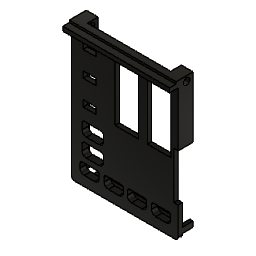
v2 - Timer - Bottom overlay (Autodesk Fusion 360 design; units mm, degrees)
Autodesk Fusion 360 part; units mm, degrees
sketch "Sketch1" plane through (0, 0, 0) normal (0, 1, 0) x (1, 0, 0)
  line L0 (0, 0) -> (50, 0)
  line L1 (50, 0) -> (50, -63)
  line L2 (50, -63) -> (0, -63)
  line L3 (0, -63) -> (0, 0)
  line L4 (20.9, -55.9) -> (31, -55.9)
  line L5 (31, -55.9) -> (31, -30.5)
  line L6 (31, -30.5) -> (20.9, -30.5)
  line L7 (20.9, -30.5) -> (20.9, -55.9)
  line L8 (36, -55.9) -> (46.1, -55.9)
  line L9 (46.1, -55.9) -> (46.1, -30.5)
  line L10 (46.1, -30.5) -> (36, -30.5)
  line L11 (36, -30.5) -> (36, -55.9)
  line L12 (0, 0) -> (50, 0)
  line L13 (50, 0) -> (50, 2)
  line L14 (50, 2) -> (0, 2)
  line L15 (0, 2) -> (0, 0)
  line L16 (6, -32.5) -> (11, -32.5)
  line L17 (11, -32.5) -> (11, -30.5)
  line L18 (11, -30.5) -> (6, -30.5)
  line L19 (6, -30.5) -> (6, -32.5)
  line L20 (6, -44.2) -> (11, -44.2)
  line L21 (11, -44.2) -> (11, -42.2)
  line L22 (11, -42.2) -> (6, -42.2)
  line L23 (6, -42.2) -> (6, -44.2)
  line L24 (6, -55.9) -> (11, -55.9)
  line L25 (11, -55.9) -> (11, -53.9)
  line L26 (11, -53.9) -> (6, -53.9)
  line L27 (6, -53.9) -> (6, -55.9)
  line L28 (13, -2.5) -> (4, -2.5)
  line L29 (4, -2.5) -> (4, -7.5)
  line L30 (4, -7.5) -> (13, -7.5)
  line L31 (13, -7.5) -> (13, -2.5)
  line L32 (13, -2.5) -> (4, -7.5) construction
  line L33 (4, -2.5) -> (13, -7.5) construction
  line L34 (24.33, -2.5) -> (15.33, -2.5)
  line L35 (15.33, -2.5) -> (15.33, -7.5)
  line L36 (15.33, -7.5) -> (24.33, -7.5)
  line L37 (24.33, -7.5) -> (24.33, -2.5)
  line L38 (24.33, -2.5) -> (15.33, -7.5) construction
  line L39 (15.33, -2.5) -> (24.33, -7.5) construction
  line L40 (35.16, -2.5) -> (26.16, -2.5)
  line L41 (26.16, -2.5) -> (26.16, -7.5)
  line L42 (26.16, -7.5) -> (35.16, -7.5)
  line L43 (35.16, -7.5) -> (35.16, -2.5)
  line L44 (35.16, -2.5) -> (26.16, -7.5) construction
  line L45 (26.16, -2.5) -> (35.16, -7.5) construction
  line L46 (46.49, -2.5) -> (37.49, -2.5)
  line L47 (37.49, -2.5) -> (37.49, -7.5)
  line L48 (37.49, -7.5) -> (46.49, -7.5)
  line L49 (46.49, -7.5) -> (46.49, -2.5)
  line L50 (46.49, -2.5) -> (37.49, -7.5) construction
  line L51 (37.49, -2.5) -> (46.49, -7.5) construction
  line L52 (7, -24.5) -> (13, -24.5)
  line L53 (13, -18.5) -> (7, -18.5)
  line L54 (15, -18.5) -> (5, -18.5)
  line L55 (5, -18.5) -> (5, -24.5)
  line L56 (5, -24.5) -> (15, -24.5)
  line L57 (15, -24.5) -> (15, -18.5)
  line L58 (15, -18.5) -> (5, -24.5) construction
  line L59 (5, -18.5) -> (15, -24.5) construction
  line L60 (15, -10) -> (5, -10)
  line L61 (5, -10) -> (5, -16)
  line L62 (5, -16) -> (15, -16)
  line L63 (15, -16) -> (15, -10)
  line L64 (15, -10) -> (5, -16) construction
  line L65 (5, -10) -> (15, -16) construction
  point P0 (8.5, -5)
  point P1 (19.83, -5)
  point P2 (30.66, -5)
  point P3 (41.99, -5)
  point P4 (10, -21.5)
  point P5 (10, -13)
  dimension "d1" = 50
  dimension "d2" = 63
  dimension "d3" = 10.1
  dimension "d4" = 25.4
  dimension "d5" = 10.1
  dimension "d6" = 25.4
  dimension "d7" = 3.9
  dimension "d8" = 5
  dimension "d9" = 30.5
  dimension "d10" = 30.5
  dimension "d19" = 2
  dimension "d58" = 5
  dimension "d59" = 2
  dimension "d60" = 6
  dimension "d61" = 30.5
  dimension "d62" = 5
  dimension "d63" = 2
  dimension "d64" = 9.7
  dimension "d65" = 5
  dimension "d66" = 2
  dimension "d67" = 9.7
  dimension "d105" = 9
  dimension "d106" = 5
  dimension "d107" = 9
  dimension "d108" = 5
  dimension "d127" = 9
  dimension "d128" = 5
  dimension "d129" = 9
  dimension "d130" = 5
  dimension "d151" = 6
  dimension "d152" = 6
  dimension "d159" = 10
  dimension "d160" = 6
  dimension "d161" = 10
  dimension "d162" = 6
  constraint horizontal L0
  constraint vertical L1
  constraint horizontal L2
  constraint vertical L3
  constraint coincident L0.start L3.end
  constraint horizontal L4
  constraint vertical L5
  constraint horizontal L6
  constraint vertical L7
  constraint horizontal L8
  constraint vertical L9
  constraint horizontal L10
  constraint vertical L11
  constraint horizontal L12
  constraint vertical L13
  constraint horizontal L14
  constraint vertical L15
  constraint horizontal L16
  constraint vertical L17
  constraint horizontal L18
  constraint vertical L19
  constraint horizontal L20
  constraint vertical L21
  constraint horizontal L22
  constraint vertical L23
  constraint horizontal L24
  constraint vertical L25
  constraint horizontal L26
  constraint vertical L27
  constraint horizontal L28
  constraint perpendicular L28 L29
  constraint parallel L28 L30
  constraint parallel L29 L31
  constraint coincident L32 P0
  constraint coincident L33 P0
  constraint horizontal L34
  constraint perpendicular L34 L35
  constraint parallel L34 L36
  constraint parallel L35 L37
  constraint coincident L38 P1
  constraint coincident L39 P1
  constraint horizontal L40
  constraint perpendicular L40 L41
  constraint parallel L40 L42
  constraint parallel L41 L43
  constraint coincident L44 P2
  constraint coincident L45 P2
  constraint horizontal L46
  constraint perpendicular L46 L47
  constraint parallel L46 L48
  constraint parallel L47 L49
  constraint coincident L50 P3
  constraint coincident L51 P3
  constraint horizontal L52
  constraint horizontal L53
  constraint horizontal L54
  constraint perpendicular L54 L55
  constraint parallel L54 L56
  constraint parallel L55 L57
  constraint coincident L58 P4
  constraint coincident L59 P4
  constraint horizontal L60
  constraint perpendicular L60 L61
  constraint parallel L60 L62
  constraint parallel L61 L63
  constraint coincident L64 P5
  constraint coincident L65 P5
  measures "d1" distance of L0.start L0.end
  measures "d2" distance of L0.start L2.end
  measures "d3" distance of L4.start L4.end
  measures "d4" distance of L4.start L6.end
  measures "d5" distance of L8.start L8.end
  measures "d6" distance of L8.start L10.end
  measures "d7" distance of L1 L9
  measures "d8" distance of L5 L11
  measures "d9" distance of L0 L10
  measures "d10" distance of L0 L6
  measures "d19" distance of L0.start L14.end
  measures "d58" distance of L16.start L16.end
  measures "d59" distance of L16.start L18.end
  measures "d60" distance of L3 L19
  measures "d61" distance of L0 L18
  measures "d62" distance of L20.start L20.end
  measures "d63" distance of L20.start L22.end
  measures "d64" distance of L16 L22
  measures "d65" distance of L24.start L24.end
  measures "d66" distance of L24.start L26.end
  measures "d67" distance of L20 L26
  measures "d105" distance of L29.end L30.end
  measures "d106" distance of L28.end L29.end
  measures "d107" distance of L35.end L36.end
  measures "d108" distance of L34.end L35.end
  measures "d127" distance of L41.end L42.end
  measures "d128" distance of L40.end L41.end
  measures "d129" distance of L47.end L48.end
  measures "d130" distance of L46.end L47.end
  measures "d151" distance of L52.start L52.end
  measures "d152" distance of L52.start L53.end
  measures "d159" distance of L55.end L56.end
  measures "d160" distance of L54.end L55.end
  measures "d161" distance of L61.end L62.end
  measures "d162" distance of L60.end L61.end
extrude "Extrude1" add sketch "Sketch1" against normal blind 2 contours L0 L1 L2 L3 L12 | L16 L17 L18 L19 | L20 L21 L22 L23 | L24 L25 L26 L27 | L28 L29 L30 L31 | L34 L35 L36 L37 | L40 L41 L42 L43 | L46 L47 L48 L49 | L52 L53 L54 L55 L56 L57 | L60 L61 L62 L63
extrude "Extrude3" add 1 faces at (16.6667, -0.6667, 0) along direction (0, 0, -1) blind 2
fillet "Fillet5" radius 1.5 1 edges at (0, -1, -2)
fillet "Fillet6" radius 1.5 1 edges at (50, -1, -2)
extrude "Extrude10" cut 1 faces at (27.6333, -0.6667, 30.5) along direction (0, 0, -1) blind 0.5
extrude "Extrude11" cut 1 faces at (31, -0.6667, 47.2667) along direction (1, 0, 0) blind 0.5
extrude "Extrude12" cut 1 faces at (42.7333, -0.6667, 30.5) along direction (0, 0, -1) blind 0.5
extrude "Extrude13" cut 1 faces at (46.1, -0.6667, 47.2667) along direction (1, 0, 0) blind 0.5
extrude "Extrude14" cut 1 faces at (20.9, -0.6667, 38.6333) along direction (-1, 0, 0) blind 0.5
extrude "Extrude15" cut 1 faces at (24.1, -1.3333, 55.9) along direction (0, 0, 1) blind 0.5
extrude "Extrude16" cut 1 faces at (39.5333, -0.6667, 55.9) along direction (0, 0, 1) blind 0.5
extrude "Extrude17" cut 1 faces at (36, -1.3333, 38.8) along direction (-1, 0, 0) blind 0.5
extrude "Extrude18" cut sketch "Sketch1" against normal blind 7 contours L16 L17 L18 L19 | L20 L21 L22 L23 | L24 L25 L26 L27
extrude "Extrude19" cut 1 faces at (7.6667, -0.6667, 55.9) along direction (0, 0, 1) blind 0.5
extrude "Extrude20" cut 1 faces at (6, -0.6667, 54.7333) along direction (-1, 0, 0) blind 0.5
extrude "Extrude21" cut 1 faces at (6, -0.6667, 42.8667) along direction (-1, 0, 0) blind 0.5
extrude "Extrude22" cut 1 faces at (7.6667, -0.6667, 32.5) along direction (0, 0, 1) blind 0.5
extrude "Extrude23" cut 1 faces at (6, -0.6667, 31.3333) along direction (-1, 0, 0) blind 0.5
extrude "Extrude24" cut 1 faces at (9.1667, -0.6667, 30.5) along direction (0, 0, -1) blind 0.5
extrude "Extrude25" cut 1 faces at (11, -1.3333, 32) along direction (1, 0, 0) blind 0.5
extrude "Extrude26" cut 1 faces at (9.1667, -0.6667, 42.2) along direction (0, 0, -1) blind 0.5
extrude "Extrude27" cut 1 faces at (11, -0.6667, 43.3667) along direction (1, 0, 0) blind 0.5
extrude "Extrude28" cut 1 faces at (9.1667, -0.6667, 53.9) along direction (0, 0, -1) blind 0.5
extrude "Extrude29" cut 1 faces at (11, -1.3333, 55.4) along direction (1, 0, 0) blind 0.5
extrude "Extrude30" cut sketch "Sketch1" against normal blind 3 contours L28 L29 L30 L31 | L34 L35 L36 L37
fillet "Fillet7" radius 1 1 edges at (4, -1, 7.5)
fillet "Fillet8" radius 1 1 edges at (13, -1, 7.5)
fillet "Fillet9" radius 2 1 edges at (13, -1, 2.5)
fillet "Fillet10" radius 2 1 edges at (4, -1, 2.5)
fillet "Fillet11" radius 1 1 edges at (15.33, -1, 7.5)
fillet "Fillet12" radius 1 1 edges at (24.33, -1, 7.5)
fillet "Fillet13" radius 2 1 edges at (24.33, -1, 2.5)
fillet "Fillet14" radius 2 1 edges at (15.33, -1, 2.5)
extrude "Extrude31" cut sketch "Sketch1" against normal blind 4 contours L40 L41 L42 L43 | L46 L47 L48 L49
fillet "Fillet15" radius 2 1 edges at (46.49, -1, 2.5)
fillet "Fillet16" radius 2 1 edges at (35.16, -1, 2.5)
fillet "Fillet17" radius 2 1 edges at (26.16, -1, 2.5)
fillet "Fillet18" radius 2 1 edges at (37.49, -1, 2.5)
fillet "Fillet19" radius 1 1 edges at (46.49, -1, 7.5)
fillet "Fillet20" radius 1 1 edges at (35.16, -1, 7.5)
fillet "Fillet21" radius 1 1 edges at (26.16, -1, 7.5)
fillet "Fillet22" radius 1 1 edges at (37.49, -1, 7.5)
extrude "Extrude32" cut 1 faces at (7.5, -1.3333, 44.2) along direction (0, 0, 1) blind 0.5
extrude "Extrude33" cut sketch "Sketch1" against normal blind 6 contours L52 L53 L54 L55 L56 L57 | L60 L61 L62 L63
fillet "Fillet23" radius 1 1 edges at (15, -1, 24.5)
fillet "Fillet24" radius 2 1 edges at (15, -1, 18.5)
fillet "Fillet25" radius 1 1 edges at (5, -1, 24.5)
fillet "Fillet26" radius 1 1 edges at (5, -1, 16)
fillet "Fillet27" radius 1 1 edges at (15, -1, 16)
fillet "Fillet28" radius 2 1 edges at (15, -1, 10)
fillet "Fillet29" radius 2 1 edges at (5, -1, 10)
fillet "Fillet30" radius 2 1 edges at (5, -1, 18.5)
sketch "Sketch2" plane through (0, 0, 0) normal (0, 1, 0) x (-1, 0, 0)
  line L0 (-7, 18.5) -> (-13, 18.5)
  arc A0 (-15, 20.5) -> (-13, 18.5) centre (-13, 20.5) ccw
  line L1 (-15, 20.5) -> (-15, 23.5)
  arc A1 (-14, 24.5) -> (-15, 23.5) centre (-14, 23.5) ccw
  line L2 (-14, 24.5) -> (-6, 24.5)
  arc A2 (-5, 23.5) -> (-6, 24.5) centre (-6, 23.5) ccw
  line L3 (-5, 23.5) -> (-5, 20.5)
  arc A3 (-7, 18.5) -> (-5, 20.5) centre (-7, 20.5) ccw
  line L4 (-7, 10) -> (-13, 10)
  arc A4 (-15, 12) -> (-13, 10) centre (-13, 12) ccw
  line L5 (-15, 12) -> (-15, 15)
  arc A5 (-14, 16) -> (-15, 15) centre (-14, 15) ccw
  line L6 (-14, 16) -> (-6, 16)
  arc A6 (-5, 15) -> (-6, 16) centre (-6, 15) ccw
  line L7 (-5, 15) -> (-5, 12)
  arc A7 (-7, 10) -> (-5, 12) centre (-7, 12) ccw
  line L8 (-5.5, 53.4) -> (-11.5, 53.4)
  line L9 (-11.5, 53.4) -> (-11.5, 56.4)
  line L10 (-11.5, 56.4) -> (-5.5, 56.4)
  line L11 (-5.5, 56.4) -> (-5.5, 53.4)
  line L12 (-11.5, 41.7) -> (-11.5, 44.7)
  line L13 (-11.5, 44.7) -> (-5.5, 44.7)
  line L14 (-5.5, 44.7) -> (-5.5, 41.7)
  line L15 (-5.5, 41.7) -> (-11.5, 41.7)
  line L16 (-5.5, 30) -> (-11.5, 30)
  line L17 (-11.5, 30) -> (-11.5, 33)
  line L18 (-11.5, 33) -> (-5.5, 33)
  line L19 (-5.5, 33) -> (-5.5, 30)
  line L20 (-46.6, 56.4) -> (-35.5, 56.4)
  line L21 (-35.5, 56.4) -> (-35.5, 30)
  line L22 (-35.5, 30) -> (-46.6, 30)
  line L23 (-46.6, 30) -> (-46.6, 56.4)
  line L24 (-31.5, 30) -> (-31.5, 56.4)
  line L25 (-31.5, 56.4) -> (-20.4, 56.4)
  line L26 (-20.4, 56.4) -> (-20.4, 30)
  line L27 (-20.4, 30) -> (-31.5, 30)
  arc A8 (-50, -0.5) -> (-48.5, -2) centre (-48.5, -0.5) ccw
  line L28 (-48.5, -2) -> (-1.5, -2)
  arc A9 (-1.5, -2) -> (0, -0.5) centre (-1.5, -0.5) ccw
  line L29 (0, -0.5) -> (0, 63)
  line L30 (0, 63) -> (-50, 63)
  line L31 (-50, 63) -> (-50, -0.5)
  line L32 (-6, 2.5) -> (-11, 2.5)
  arc A10 (-13, 4.5) -> (-11, 2.5) centre (-11, 4.5) ccw
  line L33 (-13, 4.5) -> (-13, 6.5)
  arc A11 (-12, 7.5) -> (-13, 6.5) centre (-12, 6.5) ccw
  line L34 (-12, 7.5) -> (-5, 7.5)
  arc A12 (-4, 6.5) -> (-5, 7.5) centre (-5, 6.5) ccw
  line L35 (-4, 6.5) -> (-4, 4.5)
  arc A13 (-6, 2.5) -> (-4, 4.5) centre (-6, 4.5) ccw
  line L36 (-17.33, 2.5) -> (-22.33, 2.5)
  arc A14 (-24.33, 4.5) -> (-22.33, 2.5) centre (-22.33, 4.5) ccw
  line L37 (-24.33, 4.5) -> (-24.33, 6.5)
  arc A15 (-23.33, 7.5) -> (-24.33, 6.5) centre (-23.33, 6.5) ccw
  line L38 (-23.33, 7.5) -> (-16.33, 7.5)
  arc A16 (-15.33, 6.5) -> (-16.33, 7.5) centre (-16.33, 6.5) ccw
  line L39 (-15.33, 6.5) -> (-15.33, 4.5)
  arc A17 (-17.33, 2.5) -> (-15.33, 4.5) centre (-17.33, 4.5) ccw
  line L40 (-28.16, 2.5) -> (-33.16, 2.5)
  arc A18 (-35.16, 4.5) -> (-33.16, 2.5) centre (-33.16, 4.5) ccw
  line L41 (-35.16, 4.5) -> (-35.16, 6.5)
  arc A19 (-34.16, 7.5) -> (-35.16, 6.5) centre (-34.16, 6.5) ccw
  line L42 (-34.16, 7.5) -> (-27.16, 7.5)
  arc A20 (-26.16, 6.5) -> (-27.16, 7.5) centre (-27.16, 6.5) ccw
  line L43 (-26.16, 6.5) -> (-26.16, 4.5)
  arc A21 (-28.16, 2.5) -> (-26.16, 4.5) centre (-28.16, 4.5) ccw
  line L44 (-39.49, 2.5) -> (-44.49, 2.5)
  arc A22 (-46.49, 4.5) -> (-44.49, 2.5) centre (-44.49, 4.5) ccw
  line L45 (-46.49, 4.5) -> (-46.49, 6.5)
  arc A23 (-45.49, 7.5) -> (-46.49, 6.5) centre (-45.49, 6.5) ccw
  line L46 (-45.49, 7.5) -> (-38.49, 7.5)
  arc A24 (-37.49, 6.5) -> (-38.49, 7.5) centre (-38.49, 6.5) ccw
  line L47 (-37.49, 6.5) -> (-37.49, 4.5)
  arc A25 (-39.49, 2.5) -> (-37.49, 4.5) centre (-39.49, 4.5) ccw
  line L48 (-50, 63) -> (-48.5, 63)
  line L49 (-48.5, 63) -> (-48.5, 0)
  line L50 (-48.5, 0) -> (-50, 0)
  line L51 (-50, 0) -> (-50, 63)
  line L52 (0, 63) -> (-1.5, 63)
  line L53 (-1.5, 63) -> (-1.5, 0)
  line L54 (-1.5, 0) -> (0, 0)
  line L55 (0, 0) -> (0, 63)
  dimension "d181" = 1.5
  dimension "d182" = 63
  dimension "d183" = 1.5
  dimension "d184" = 63
  constraint horizontal L48
  constraint vertical L49
  constraint horizontal L50
  constraint vertical L51
  constraint coincident L30.end L31.start
  constraint horizontal L52
  constraint vertical L53
  constraint horizontal L54
  constraint vertical L55
  constraint coincident L29.end L30.start
  measures "d181" distance of L30.end L48.end
  measures "d182" distance of L30.end L50.end
  measures "d183" distance of L29.end L52.end
  measures "d184" distance of L29.end L54.end
extrude "Extrude34" add sketch "Sketch2" along normal blind 3 contours L30 L31 L48 L49 L50 L51 | L29 L30 L52 L53 L54 L55
extrude "Extrude35" add 2 faces at (49.5, 3, 42) (0.5, 3, 21) along direction (0, 1, 0) blind 2
sketch "Sketch3" plane through (50, 0, 0) normal (1, 0, 0) x (0, 1, 0)
  line L0 (-2, -0.5) -> (0, -0.5)
  line L1 (0, -0.5) -> (0, 0)
  line L2 (0, 0) -> (5, 0)
  line L3 (5, 0) -> (5, 63)
  line L4 (5, 63) -> (-2, 63)
  line L5 (-2, 63) -> (-2, -0.5)
  circle A0 centre (2, 60.7) radius 1.5
  dimension "d189" = 2.3
  dimension "d190" = 3
  dimension "d203" = 3
  measures "d189" distance of L4 A0.centre
  measures "d190" distance of L3 A0.centre
  measures "d203" diameter of A0
extrude "Extrude36" cut sketch "Sketch3" against normal blind 50 contours A0
sketch "Sketch4" plane through (48.5, 0, 0) normal (-1, 0, 0) x (0, -1, 0)
  circle A0 centre (-2, 60.7) radius 1.5
  line L0 (0, 0) -> (0, 63)
  line L1 (0, 63) -> (-5, 63)
  line L2 (-5, 63) -> (-5, 0)
  line L3 (-5, 0) -> (0, 0)
sketch "Sketch5" plane through (0, -2, 0) normal (0, -1, 0) x (1, 0, 0)
  line L0 (13, 18.5) -> (7, 18.5)
  arc A0 (5, 20.5) -> (7, 18.5) centre (7, 20.5) ccw
  line L1 (5, 20.5) -> (5, 23.5)
  arc A1 (6, 24.5) -> (5, 23.5) centre (6, 23.5) ccw
  line L2 (6, 24.5) -> (14, 24.5)
  arc A2 (15, 23.5) -> (14, 24.5) centre (14, 23.5) ccw
  line L3 (15, 23.5) -> (15, 20.5)
  arc A3 (13, 18.5) -> (15, 20.5) centre (13, 20.5) ccw
  line L4 (13, 10) -> (7, 10)
  arc A4 (5, 12) -> (7, 10) centre (7, 12) ccw
  line L5 (5, 12) -> (5, 15)
  arc A5 (6, 16) -> (5, 15) centre (6, 15) ccw
  line L6 (6, 16) -> (14, 16)
  arc A6 (15, 15) -> (14, 16) centre (14, 15) ccw
  line L7 (15, 15) -> (15, 12)
  arc A7 (13, 10) -> (15, 12) centre (13, 12) ccw
  line L8 (11.5, 44.7) -> (11.5, 41.7)
  line L9 (11.5, 41.7) -> (5.5, 41.7)
  line L10 (5.5, 41.7) -> (5.5, 44.7)
  line L11 (5.5, 44.7) -> (11.5, 44.7)
  line L12 (44.49, 2.5) -> (39.49, 2.5)
  arc A8 (37.49, 4.5) -> (39.49, 2.5) centre (39.49, 4.5) ccw
  line L13 (37.49, 4.5) -> (37.49, 6.5)
  arc A9 (38.49, 7.5) -> (37.49, 6.5) centre (38.49, 6.5) ccw
  line L14 (38.49, 7.5) -> (45.49, 7.5)
  arc A10 (46.49, 6.5) -> (45.49, 7.5) centre (45.49, 6.5) ccw
  line L15 (46.49, 6.5) -> (46.49, 4.5)
  arc A11 (44.49, 2.5) -> (46.49, 4.5) centre (44.49, 4.5) ccw
  line L16 (33.16, 2.5) -> (28.16, 2.5)
  arc A12 (26.16, 4.5) -> (28.16, 2.5) centre (28.16, 4.5) ccw
  line L17 (26.16, 4.5) -> (26.16, 6.5)
  arc A13 (27.16, 7.5) -> (26.16, 6.5) centre (27.16, 6.5) ccw
  line L18 (27.16, 7.5) -> (34.16, 7.5)
  arc A14 (35.16, 6.5) -> (34.16, 7.5) centre (34.16, 6.5) ccw
  line L19 (35.16, 6.5) -> (35.16, 4.5)
  arc A15 (33.16, 2.5) -> (35.16, 4.5) centre (33.16, 4.5) ccw
  line L20 (22.33, 2.5) -> (17.33, 2.5)
  arc A16 (15.33, 4.5) -> (17.33, 2.5) centre (17.33, 4.5) ccw
  line L21 (15.33, 4.5) -> (15.33, 6.5)
  arc A17 (16.33, 7.5) -> (15.33, 6.5) centre (16.33, 6.5) ccw
  line L22 (16.33, 7.5) -> (23.33, 7.5)
  arc A18 (24.33, 6.5) -> (23.33, 7.5) centre (23.33, 6.5) ccw
  line L23 (24.33, 6.5) -> (24.33, 4.5)
  arc A19 (22.33, 2.5) -> (24.33, 4.5) centre (22.33, 4.5) ccw
  line L24 (11, 2.5) -> (6, 2.5)
  arc A20 (4, 4.5) -> (6, 2.5) centre (6, 4.5) ccw
  line L25 (4, 4.5) -> (4, 6.5)
  arc A21 (5, 7.5) -> (4, 6.5) centre (5, 6.5) ccw
  line L26 (5, 7.5) -> (12, 7.5)
  arc A22 (13, 6.5) -> (12, 7.5) centre (12, 6.5) ccw
  line L27 (13, 6.5) -> (13, 4.5)
  arc A23 (11, 2.5) -> (13, 4.5) centre (11, 4.5) ccw
  line L28 (11.5, 53.4) -> (5.5, 53.4)
  line L29 (5.5, 53.4) -> (5.5, 56.4)
  line L30 (5.5, 56.4) -> (11.5, 56.4)
  line L31 (11.5, 56.4) -> (11.5, 53.4)
  line L32 (11.5, 30) -> (5.5, 30)
  line L33 (5.5, 30) -> (5.5, 33)
  line L34 (5.5, 33) -> (11.5, 33)
  line L35 (11.5, 33) -> (11.5, 30)
  line L36 (35.5, 56.4) -> (46.6, 56.4)
  line L37 (46.6, 56.4) -> (46.6, 30)
  line L38 (46.6, 30) -> (35.5, 30)
  line L39 (35.5, 30) -> (35.5, 56.4)
  line L40 (31.5, 56.4) -> (31.5, 30)
  line L41 (31.5, 30) -> (20.4, 30)
  line L42 (20.4, 30) -> (20.4, 56.4)
  line L43 (20.4, 56.4) -> (31.5, 56.4)
  arc A24 (48.5, -2) -> (50, -0.5) centre (48.5, -0.5) ccw
  line L44 (50, -0.5) -> (50, 63)
  line L45 (50, 63) -> (0, 63)
  line L46 (0, 63) -> (0, -0.5)
  arc A25 (0, -0.5) -> (1.5, -2) centre (1.5, -0.5) ccw
  line L47 (1.5, -2) -> (48.5, -2)
  line L48 (0, 63) -> (50, 63)
  line L49 (50, 63) -> (50, 61)
  line L50 (50, 61) -> (0, 61)
  line L51 (0, 61) -> (0, 63)
  line L52 (0, 61) -> (50, 61)
  line L53 (50, 61) -> (50, 62)
  line L54 (50, 62) -> (0, 62)
  line L55 (0, 62) -> (0, 61)
  constraint horizontal L48
  constraint vertical L49
  constraint horizontal L50
  constraint vertical L51
  constraint coincident L44 L49.end
  constraint coincident L45.end L46.start
  constraint horizontal L52
  constraint vertical L53
  constraint horizontal L54
  constraint vertical L55
  constraint midpoint L49 L53.end
extrude "Extrude37" add sketch "Sketch5" along normal blind 3 contours L44 L46 L49 L50 L51 L52 L53 L54 L55
extrude "Extrude38" add 1 faces at (16.6667, -5, 61.3333) along direction (0, -1, 0) blind 1
extrude "Extrude39" add 1 faces at (33.3333, -4.6667, 61) along direction (0, 0, -1) blind 1
extrude "Extrude40" add 1 faces at (33.3333, -2, 62.3333) along direction (0, -1, 0) blind 1
sketch "Sketch6" plane through (1.5, 0, 0) normal (1, 0, 0) x (0, 1, 0)
  circle A0 centre (2, 60.7) radius 1.5
  line L0 (0, 63) -> (0, 0)
  line L1 (0, 0) -> (5, 0)
  line L2 (5, 0) -> (5, 63)
  line L3 (5, 63) -> (0, 63)
  line L4 (5, 63) -> (0, 63)
  line L5 (0, 63) -> (0, 58)
  line L6 (0, 58) -> (5, 58)
  line L7 (5, 58) -> (5, 63)
  dimension "d204" = 5
  constraint horizontal L4
  constraint vertical L5
  constraint horizontal L6
  constraint vertical L7
  constraint coincident L0 L5.end
  constraint coincident L2.end L3.start
  measures "d204" distance of L2.end L6.end
extrude "Extrude42" add sketch "Sketch6" along normal blind 48 contours L0 L2 L3 L4 L5 L6 L7
sketch "Sketch7" plane through (0, 5, 0) normal (0, 1, 0) x (-1, 0, 0)
  line L0 (0, 0) -> (0, 63)
  line L1 (0, 63) -> (-50, 63)
  line L2 (-50, 63) -> (-50, 0)
  line L3 (-50, 0) -> (-48.5, 0)
  line L4 (-48.5, 0) -> (-48.5, 58)
  line L5 (-48.5, 58) -> (-1.5, 58)
  line L6 (-1.5, 58) -> (-1.5, 0)
  line L7 (-1.5, 0) -> (0, 0)
  line L8 (-48.5, 58) -> (-1.5, 58)
  line L9 (-1.5, 58) -> (-1.5, 63)
  line L10 (-1.5, 63) -> (-48.5, 63)
  line L11 (-48.5, 63) -> (-48.5, 58)
  line L12 (-48.5, 58) -> (-44.5, 58)
  line L13 (-44.5, 58) -> (-44.5, 63)
  line L14 (-44.5, 63) -> (-48.5, 63)
  line L15 (-48.5, 63) -> (-48.5, 58)
  line L16 (-1.5, 58) -> (-5.5, 58)
  line L17 (-5.5, 58) -> (-5.5, 63)
  line L18 (-5.5, 63) -> (-1.5, 63)
  line L19 (-1.5, 63) -> (-1.5, 58)
  dimension "d207" = 4
  dimension "d208" = 4
  dimension "d209" = 5
  constraint horizontal L8
  constraint vertical L9
  constraint horizontal L10
  constraint vertical L11
  constraint coincident L1 L9.end
  constraint coincident L4.end L5.start
  constraint horizontal L12
  constraint vertical L13
  constraint horizontal L14
  constraint vertical L15
  constraint horizontal L16
  constraint vertical L17
  constraint horizontal L18
  constraint vertical L19
  constraint coincident L5.end L6.start
  measures "d207" distance of L4.end L12.end
  measures "d208" distance of L5.end L16.end
  measures "d209" distance of L5.end L9.end
extrude "Extrude43" cut sketch "Sketch7" against normal blind 5 contours L1 L5 L8 L10 L13 L17
sketch "Sketch8" plane through (0, 0, 0) normal (0, 1, 0) x (-1, 0, 0)
  line L0 (-7, 18.5) -> (-13, 18.5)
  arc A0 (-15, 20.5) -> (-13, 18.5) centre (-13, 20.5) ccw
  line L1 (-15, 20.5) -> (-15, 23.5)
  arc A1 (-14, 24.5) -> (-15, 23.5) centre (-14, 23.5) ccw
  line L2 (-14, 24.5) -> (-6, 24.5)
  arc A2 (-5, 23.5) -> (-6, 24.5) centre (-6, 23.5) ccw
  line L3 (-5, 23.5) -> (-5, 20.5)
  arc A3 (-7, 18.5) -> (-5, 20.5) centre (-7, 20.5) ccw
  line L4 (-7, 10) -> (-13, 10)
  arc A4 (-15, 12) -> (-13, 10) centre (-13, 12) ccw
  line L5 (-15, 12) -> (-15, 15)
  arc A5 (-14, 16) -> (-15, 15) centre (-14, 15) ccw
  line L6 (-14, 16) -> (-6, 16)
  arc A6 (-5, 15) -> (-6, 16) centre (-6, 15) ccw
  line L7 (-5, 15) -> (-5, 12)
  arc A7 (-7, 10) -> (-5, 12) centre (-7, 12) ccw
  line L8 (-5.5, 53.4) -> (-11.5, 53.4)
  line L9 (-11.5, 53.4) -> (-11.5, 56.4)
  line L10 (-11.5, 56.4) -> (-5.5, 56.4)
  line L11 (-5.5, 56.4) -> (-5.5, 53.4)
  line L12 (-11.5, 41.7) -> (-11.5, 44.7)
  line L13 (-11.5, 44.7) -> (-5.5, 44.7)
  line L14 (-5.5, 44.7) -> (-5.5, 41.7)
  line L15 (-5.5, 41.7) -> (-11.5, 41.7)
  line L16 (-5.5, 30) -> (-11.5, 30)
  line L17 (-11.5, 30) -> (-11.5, 33)
  line L18 (-11.5, 33) -> (-5.5, 33)
  line L19 (-5.5, 33) -> (-5.5, 30)
  line L20 (-46.6, 56.4) -> (-35.5, 56.4)
  line L21 (-35.5, 56.4) -> (-35.5, 30)
  line L22 (-35.5, 30) -> (-46.6, 30)
  line L23 (-46.6, 30) -> (-46.6, 56.4)
  line L24 (-31.5, 30) -> (-31.5, 56.4)
  line L25 (-31.5, 56.4) -> (-20.4, 56.4)
  line L26 (-20.4, 56.4) -> (-20.4, 30)
  line L27 (-20.4, 30) -> (-31.5, 30)
  line L28 (-6, 2.5) -> (-11, 2.5)
  arc A8 (-13, 4.5) -> (-11, 2.5) centre (-11, 4.5) ccw
  line L29 (-13, 4.5) -> (-13, 6.5)
  arc A9 (-12, 7.5) -> (-13, 6.5) centre (-12, 6.5) ccw
  line L30 (-12, 7.5) -> (-5, 7.5)
  arc A10 (-4, 6.5) -> (-5, 7.5) centre (-5, 6.5) ccw
  line L31 (-4, 6.5) -> (-4, 4.5)
  arc A11 (-6, 2.5) -> (-4, 4.5) centre (-6, 4.5) ccw
  line L32 (-17.33, 2.5) -> (-22.33, 2.5)
  arc A12 (-24.33, 4.5) -> (-22.33, 2.5) centre (-22.33, 4.5) ccw
  line L33 (-24.33, 4.5) -> (-24.33, 6.5)
  arc A13 (-23.33, 7.5) -> (-24.33, 6.5) centre (-23.33, 6.5) ccw
  line L34 (-23.33, 7.5) -> (-16.33, 7.5)
  arc A14 (-15.33, 6.5) -> (-16.33, 7.5) centre (-16.33, 6.5) ccw
  line L35 (-15.33, 6.5) -> (-15.33, 4.5)
  arc A15 (-17.33, 2.5) -> (-15.33, 4.5) centre (-17.33, 4.5) ccw
  line L36 (-28.16, 2.5) -> (-33.16, 2.5)
  arc A16 (-35.16, 4.5) -> (-33.16, 2.5) centre (-33.16, 4.5) ccw
  line L37 (-35.16, 4.5) -> (-35.16, 6.5)
  arc A17 (-34.16, 7.5) -> (-35.16, 6.5) centre (-34.16, 6.5) ccw
  line L38 (-34.16, 7.5) -> (-27.16, 7.5)
  arc A18 (-26.16, 6.5) -> (-27.16, 7.5) centre (-27.16, 6.5) ccw
  line L39 (-26.16, 6.5) -> (-26.16, 4.5)
  arc A19 (-28.16, 2.5) -> (-26.16, 4.5) centre (-28.16, 4.5) ccw
  line L40 (-39.49, 2.5) -> (-44.49, 2.5)
  arc A20 (-46.49, 4.5) -> (-44.49, 2.5) centre (-44.49, 4.5) ccw
  line L41 (-46.49, 4.5) -> (-46.49, 6.5)
  arc A21 (-45.49, 7.5) -> (-46.49, 6.5) centre (-45.49, 6.5) ccw
  line L42 (-45.49, 7.5) -> (-38.49, 7.5)
  arc A22 (-37.49, 6.5) -> (-38.49, 7.5) centre (-38.49, 6.5) ccw
  line L43 (-37.49, 6.5) -> (-37.49, 4.5)
  arc A23 (-39.49, 2.5) -> (-37.49, 4.5) centre (-39.49, 4.5) ccw
  line L44 (-1.5, 58) -> (-5.5, 58)
  line L45 (-5.5, 58) -> (-5.5, 63)
  line L46 (-5.5, 63) -> (-44.5, 63)
  line L47 (-44.5, 63) -> (-44.5, 58)
  line L48 (-44.5, 58) -> (-48.5, 58)
  line L49 (-48.5, 58) -> (-48.5, 0)
  line L50 (-48.5, 0) -> (-50, 0)
  line L51 (-50, 0) -> (-50, -0.5)
  arc A24 (-50, -0.5) -> (-48.5, -2) centre (-48.5, -0.5) ccw
  line L52 (-48.5, -2) -> (-1.5, -2)
  arc A25 (-1.5, -2) -> (0, -0.5) centre (-1.5, -0.5) ccw
  line L53 (0, -0.5) -> (0, 0)
  line L54 (0, 0) -> (-1.5, 0)
  line L55 (-1.5, 0) -> (-1.5, 58)
  arc A26 (-47.99, 4.5) -> (-44.49, 1) centre (-44.49, 4.5) ccw
  line L56 (-39.49, 1) -> (-44.49, 1)
  arc A27 (-39.49, 1) -> (-35.99, 4.5) centre (-39.49, 4.5) ccw
  line L57 (-35.99, 6.5) -> (-35.99, 4.5)
  arc A28 (-35.99, 6.5) -> (-38.49, 9) centre (-38.49, 6.5) ccw
  line L58 (-45.49, 9) -> (-38.49, 9)
  arc A29 (-45.49, 9) -> (-47.99, 6.5) centre (-45.49, 6.5) ccw
  line L59 (-47.99, 4.5) -> (-47.99, 6.5)
  arc A30 (-24.66, 6.5) -> (-27.16, 9) centre (-27.16, 6.5) ccw
  line L60 (-34.16, 9) -> (-27.16, 9)
  arc A31 (-34.16, 9) -> (-36.66, 6.5) centre (-34.16, 6.5) ccw
  line L61 (-36.66, 4.5) -> (-36.66, 6.5)
  arc A32 (-36.66, 4.5) -> (-33.16, 1) centre (-33.16, 4.5) ccw
  line L62 (-28.16, 1) -> (-33.16, 1)
  arc A33 (-28.16, 1) -> (-24.66, 4.5) centre (-28.16, 4.5) ccw
  line L63 (-24.66, 6.5) -> (-24.66, 4.5)
  arc A34 (-13.83, 6.5) -> (-16.33, 9) centre (-16.33, 6.5) ccw
  line L64 (-23.33, 9) -> (-16.33, 9)
  arc A35 (-23.33, 9) -> (-25.83, 6.5) centre (-23.33, 6.5) ccw
  line L65 (-25.83, 4.5) -> (-25.83, 6.5)
  arc A36 (-25.83, 4.5) -> (-22.33, 1) centre (-22.33, 4.5) ccw
  line L66 (-17.33, 1) -> (-22.33, 1)
  arc A37 (-17.33, 1) -> (-13.83, 4.5) centre (-17.33, 4.5) ccw
  line L67 (-13.83, 6.5) -> (-13.83, 4.5)
  arc A38 (-2.5, 6.5) -> (-5, 9) centre (-5, 6.5) ccw
  line L68 (-12, 9) -> (-5, 9)
  arc A39 (-12, 9) -> (-14.5, 6.5) centre (-12, 6.5) ccw
  line L69 (-14.5, 4.5) -> (-14.5, 6.5)
  arc A40 (-14.5, 4.5) -> (-11, 1) centre (-11, 4.5) ccw
  line L70 (-6, 1) -> (-11, 1)
  arc A41 (-6, 1) -> (-2.5, 4.5) centre (-6, 4.5) ccw
  line L71 (-2.5, 6.5) -> (-2.5, 4.5)
  arc A42 (-3.5, 15) -> (-6, 17.5) centre (-6, 15) ccw
  line L72 (-14, 17.5) -> (-6, 17.5)
  arc A43 (-14, 17.5) -> (-16.5, 15) centre (-14, 15) ccw
  line L73 (-16.5, 12) -> (-16.5, 15)
  arc A44 (-16.5, 12) -> (-13, 8.5) centre (-13, 12) ccw
  line L74 (-7, 8.5) -> (-13, 8.5)
  arc A45 (-7, 8.5) -> (-3.5, 12) centre (-7, 12) ccw
  line L75 (-3.5, 15) -> (-3.5, 12)
  arc A46 (-3.5, 23.5) -> (-6, 26) centre (-6, 23.5) ccw
  line L76 (-14, 26) -> (-6, 26)
  arc A47 (-14, 26) -> (-16.5, 23.5) centre (-14, 23.5) ccw
  line L77 (-16.5, 20.5) -> (-16.5, 23.5)
  arc A48 (-16.5, 20.5) -> (-13, 17) centre (-13, 20.5) ccw
  line L78 (-7, 17) -> (-13, 17)
  arc A49 (-7, 17) -> (-3.5, 20.5) centre (-7, 20.5) ccw
  line L79 (-3.5, 23.5) -> (-3.5, 20.5)
  dimension "d212" = -1.5
  dimension "d213" = -1.5
  dimension "d214" = -1.5
  dimension "d215" = -1.5
  dimension "d216" = -1.5
  dimension "d217" = -1.5
extrude "Extrude44" add sketch "Sketch8" along normal blind 3 contours A26 L56 A27 A28 L58 A29 L59 A31 L61 A32 | A27 L57 A28 A31 L61 A32 | A27 L57 A28 A30 L60 A31 A32 L62 A33 A35 L65 A36 | A30 A33 L63 A35 L65 A36 | A30 A33 L63 A34 L64 A35 A36 L66 A37 A39 L69 A40 | A34 A37 L67 A39 L69 A40 | A34 A37 L67 A38 L68 A39 A40 L70 A41 L71 A44 L74 A45 | L68 A39 A42 A43 L73 A44 A45 L75 A48 L78 A49 | L68 A39 A44 L74 A45 | A42 L72 A43 A46 L76 A47 L77 A48 A49 L79 | A42 L72 A43 A48 L78 A49
sketch "Sketch9" plane through (48.5, 0, 0) normal (-1, 0, 0) x (0, -1, 0)
  line L0 (0, 58) -> (-5, 58)
  line L1 (-5, 58) -> (-5, 0)
  line L2 (-5, 0) -> (0, 0)
  line L3 (0, 0) -> (0, 58)
  line L4 (0, 34.5) -> (-5, 34.5)
  line L5 (-5, 34.5) -> (-5, 12.5)
  line L6 (-5, 12.5) -> (0, 12.5)
  line L7 (0, 12.5) -> (0, 34.5)
  dimension "d220" = 22
  dimension "d221" = 12.5
  constraint horizontal L4
  constraint vertical L5
  constraint horizontal L6
  constraint vertical L7
  constraint coincident L1 L5.end
  constraint coincident L3 L4.start
  measures "d220" distance of L4 L6
  measures "d221" distance of L2 L6
extrude "Extrude45" cut sketch "Sketch9" against normal blind 8 contours L1 L3 L4 L5 L6 L7
sketch "Sketch10" plane through (50, 0, 0) normal (1, 0, 0) x (0, 1, 0)
  line L0 (5, 12.5) -> (0, 12.5)
  line L1 (0, 12.5) -> (0, 34.5)
  line L2 (0, 34.5) -> (5, 34.5)
  line L3 (5, 34.5) -> (5, 63)
  line L4 (5, 63) -> (-3, 63)
  line L5 (-3, 63) -> (-3, 62)
  line L6 (-3, 62) -> (-6, 62)
  line L7 (-6, 62) -> (-6, 60)
  line L8 (-6, 60) -> (-2, 60)
  line L9 (-2, 60) -> (-2, -0.5)
  line L10 (-2, -0.5) -> (0, -0.5)
  line L11 (0, -0.5) -> (0, 0)
  line L12 (0, 0) -> (5, 0)
  line L13 (5, 0) -> (5, 12.5)
  circle A0 centre (2, 60.7) radius 1.5
  line L14 (0, 12.5) -> (-2, 12.5)
  line L15 (-2, 12.5) -> (-2, 34.5)
  line L16 (-2, 34.5) -> (0, 34.5)
  line L17 (0, 34.5) -> (0, 12.5)
  dimension "d224" = 22
  constraint horizontal L14
  constraint vertical L15
  constraint horizontal L16
  constraint vertical L17
  constraint coincident L9 L15.end
  constraint coincident L0.end L1.start
  measures "d224" distance of L14 L16
extrude "Extrude46" cut sketch "Sketch10" against normal blind 2 contours L1 L9 L14 L15 L16 L17
sketch "Sketch11" plane through (0, 5, 0) normal (0, 1, 0) x (-1, 0, 0)
  line L0 (-48.5, 12.5) -> (-50, 12.5)
  line L1 (-50, 12.5) -> (-50, 0)
  line L2 (-50, 0) -> (-48.5, 0)
  line L3 (-48.5, 0) -> (-48.5, 12.5)
  line L4 (-50, 2.5304) -> (-48.5, 2.5304)
  line L5 (-48.5, 2.5304) -> (-48.5, 12.5)
  line L6 (-48.5, 12.5) -> (-50, 12.5)
  line L7 (-50, 12.5) -> (-50, 2.5304)
  constraint horizontal L4
  constraint vertical L5
  constraint horizontal L6
  constraint vertical L7
  constraint coincident L0.start L3.end
  constraint coincident L1 L4.start
extrude "Extrude47" cut sketch "Sketch11" against normal blind 5 contours L0 L1 L3 L4 L5 L6 L7
sketch "Sketch12" plane through (0, 0, 0) normal (0, 1, 0) x (-1, 0, 0)
  line L0 (-48, 12.5) -> (-50, 12.5)
  line L1 (-50, 12.5) -> (-50, 2.5304)
  line L2 (-50, 2.5304) -> (-48.5, 2.5304)
  line L3 (-48.5, 2.5304) -> (-48.5, 0)
  line L4 (-48.5, 0) -> (-50, 0)
  line L5 (-50, 0) -> (-50, -0.5)
  arc A0 (-50, -0.5) -> (-48.5, -2) centre (-48.5, -0.5) ccw
  line L6 (-48.5, -2) -> (-1.5, -2)
  arc A1 (-1.5, -2) -> (0, -0.5) centre (-1.5, -0.5) ccw
  line L7 (0, -0.5) -> (0, 0)
  line L8 (0, 0) -> (-1.5, 0)
  line L9 (-1.5, 0) -> (-1.5, 58)
  line L10 (-1.5, 58) -> (-5.5, 58)
  line L11 (-5.5, 58) -> (-5.5, 63)
  line L12 (-5.5, 63) -> (-44.5, 63)
  line L13 (-44.5, 63) -> (-44.5, 58)
  line L14 (-44.5, 58) -> (-48.5, 58)
  line L15 (-48.5, 58) -> (-48.5, 34.5)
  line L16 (-48.5, 34.5) -> (-48, 34.5)
  line L17 (-48, 34.5) -> (-48, 12.5)
  line L18 (-14, 26) -> (-6, 26)
  arc A2 (-3.5, 23.5) -> (-6, 26) centre (-6, 23.5) ccw
  line L19 (-3.5, 23.5) -> (-3.5, 20.5)
  arc A3 (-5.3491, 17.4138) -> (-3.5, 20.5) centre (-7, 20.5) ccw
  arc A4 (-3.5, 15) -> (-5.3491, 17.4138) centre (-6, 15) ccw
  line L20 (-3.5, 15) -> (-3.5, 12)
  arc A5 (-5.1972, 9) -> (-3.5, 12) centre (-7, 12) ccw
  line L21 (-5.1972, 9) -> (-5, 9)
  arc A6 (-2.5, 6.5) -> (-5, 9) centre (-5, 6.5) ccw
  line L22 (-2.5, 6.5) -> (-2.5, 4.5)
  arc A7 (-6, 1) -> (-2.5, 4.5) centre (-6, 4.5) ccw
  line L23 (-6, 1) -> (-11, 1)
  arc A8 (-14.165, 3.0058) -> (-11, 1) centre (-11, 4.5) ccw
  arc A9 (-17.33, 1) -> (-14.165, 3.0058) centre (-17.33, 4.5) ccw
  line L24 (-17.33, 1) -> (-22.33, 1)
  arc A10 (-25.245, 2.5628) -> (-22.33, 1) centre (-22.33, 4.5) ccw
  arc A11 (-28.16, 1) -> (-25.245, 2.5628) centre (-28.16, 4.5) ccw
  line L25 (-28.16, 1) -> (-33.16, 1)
  arc A12 (-36.325, 3.0058) -> (-33.16, 1) centre (-33.16, 4.5) ccw
  arc A13 (-39.49, 1) -> (-36.325, 3.0058) centre (-39.49, 4.5) ccw
  line L26 (-39.49, 1) -> (-44.49, 1)
  arc A14 (-47.99, 4.5) -> (-44.49, 1) centre (-44.49, 4.5) ccw
  line L27 (-47.99, 4.5) -> (-47.99, 6.5)
  arc A15 (-45.49, 9) -> (-47.99, 6.5) centre (-45.49, 6.5) ccw
  line L28 (-45.49, 9) -> (-38.49, 9)
  arc A16 (-36.325, 7.7501) -> (-38.49, 9) centre (-38.49, 6.5) ccw
  arc A17 (-34.16, 9) -> (-36.325, 7.7501) centre (-34.16, 6.5) ccw
  line L29 (-34.16, 9) -> (-27.16, 9)
  arc A18 (-25.245, 8.1071) -> (-27.16, 9) centre (-27.16, 6.5) ccw
  arc A19 (-23.33, 9) -> (-25.245, 8.1071) centre (-23.33, 6.5) ccw
  line L30 (-23.33, 9) -> (-16.33, 9)
  arc A20 (-14.165, 7.7501) -> (-16.33, 9) centre (-16.33, 6.5) ccw
  arc A21 (-13.4589, 8.5302) -> (-14.165, 7.7501) centre (-12, 6.5) ccw
  arc A22 (-16.5, 12) -> (-13.4589, 8.5302) centre (-13, 12) ccw
  line L31 (-16.5, 12) -> (-16.5, 15)
  arc A23 (-14.6509, 17.4138) -> (-16.5, 15) centre (-14, 15) ccw
  arc A24 (-16.5, 20.5) -> (-14.6509, 17.4138) centre (-13, 20.5) ccw
  line L32 (-16.5, 20.5) -> (-16.5, 23.5)
  arc A25 (-14, 26) -> (-16.5, 23.5) centre (-14, 23.5) ccw
  line L33 (-5.5, 53.4) -> (-11.5, 53.4)
  line L34 (-11.5, 53.4) -> (-11.5, 56.4)
  line L35 (-11.5, 56.4) -> (-5.5, 56.4)
  line L36 (-5.5, 56.4) -> (-5.5, 53.4)
  line L37 (-11.5, 41.7) -> (-11.5, 44.7)
  line L38 (-11.5, 44.7) -> (-5.5, 44.7)
  line L39 (-5.5, 44.7) -> (-5.5, 41.7)
  line L40 (-5.5, 41.7) -> (-11.5, 41.7)
  line L41 (-5.5, 30) -> (-11.5, 30)
  line L42 (-11.5, 30) -> (-11.5, 33)
  line L43 (-11.5, 33) -> (-5.5, 33)
  line L44 (-5.5, 33) -> (-5.5, 30)
  line L45 (-46.6, 56.4) -> (-35.5, 56.4)
  line L46 (-35.5, 56.4) -> (-35.5, 30)
  line L47 (-35.5, 30) -> (-46.6, 30)
  line L48 (-46.6, 30) -> (-46.6, 56.4)
  line L49 (-31.5, 30) -> (-31.5, 56.4)
  line L50 (-31.5, 56.4) -> (-20.4, 56.4)
  line L51 (-20.4, 56.4) -> (-20.4, 30)
  line L52 (-20.4, 30) -> (-31.5, 30)
  line L53 (-5, -2) -> (-45, -2)
  line L54 (-45, -2) -> (-45, 0)
  line L55 (-45, 0) -> (-5, 0)
  line L56 (-5, 0) -> (-5, -2)
  dimension "d229" = 40
  dimension "d230" = 2
  dimension "d231" = 5
  constraint horizontal L53
  constraint vertical L54
  constraint horizontal L55
  constraint vertical L56
  constraint coincident L6 L53.start
  measures "d229" distance of L53.start L53.end
  measures "d230" distance of L53.start L55.end
  measures "d231" distance of L7.end L56
extrude "Extrude48" add sketch "Sketch12" along normal blind 5 contours L6 L53 L54 L55 L56
extrude "Extrude49" cut 1 faces at (8, 3, 8.3333) along direction (0, -1, 0) blind 2
extrude "Extrude41" [suppressed]
